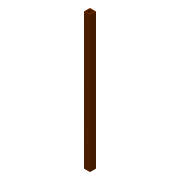
# Autodesk Inventor part: ClawArmBeam
Saved by Autodesk Inventor 2015 (Build 190159000, 159)
## iProperties
Created: 2015-01-13
Part Number: ClawArmBeam
Material: Generic
Document SubType Name: Modeling
Designer: Collin_2
Density: 1 g/cm^3
Appearance: Default
Author: Collin_2
Autodesk Inventor part; units mm, degrees
ref_plane "YZ Plane" through (0, 0, 0) normal (1, 0, 0) x (0, 1, 0)
ref_plane "XZ Plane" through (0, 0, 0) normal (0, 1, 0) x (-1, 0, 0)
ref_plane "XY Plane" through (0, 0, 0) normal (0, 0, 1) x (1, 0, 0)
sketch "Sketch1" plane through (0, 0, 0) normal (0, 1, 0) x (-1, 0, 0)
  line L0 (13.4736, 15.4721) -> (-11.9264, 15.4721)
  line L1 (-11.9264, 15.4721) -> (-11.9264, -9.9279)
  line L2 (-11.9264, -9.9279) -> (13.4736, -9.9279)
  line L3 (13.4736, -9.9279) -> (13.4736, 15.4721)
  point P0 (0, 0)
  dimension "d0" = 25.4
  dimension "d1" = 25.4
  constraints: 8 end point, 2 parallel, 1 horizontal, 1 perpendicular
  measures "d0" distance of L2.end L0.start
  measures "d1" distance of L1.end L2.end
extrude "Extrusion1" add sketch "Sketch1" along normal blind 609.6
shell "Shell1" thickness 3.175 removed faces 1 at (3.4597, 609.6, 7.0054)
sketch "Sketch2" plane through (0, 609.6, 0) normal (0, 1, 0) x (1, 0, 0)
  line L0 (-10.2986, -12.2971) -> (8.7514, -12.2971)
  line L1 (8.7514, -12.2971) -> (8.7514, 6.7529)
  line L2 (8.7514, 6.7529) -> (-10.2986, 6.7529)
  line L3 (-10.2986, 6.7529) -> (-10.2986, -12.2971)
  point P0 (0, 0)
  constraints: 8 end point, 2 parallel, 1 horizontal, 1 perpendicular
extrude "Extrusion2" cut sketch "Sketch2" against normal blind 609.6
sketch "Sketch3" plane through (-13.4736, 0, 15.4721) normal (0, 0, 1) x (1, 0, 0)
  line L0 (38.1, 608.6348) -> (0, 608.6348)
  circle A0 centre (12.7, 12.7) radius 3.3655
  circle A1 centre (12.7, 342.9) radius 3.3655
  circle A2 centre (12.7, 595.9348) radius 3.3655
  line L1 (0, 557.8348) -> (0, 608.6348)
  line L2 (0, 50.8) -> (0, 0)
  line L3 (12.7, 342.9) -> (0, 304.3174) construction
  line L4 (0, 317.5) -> (0, 368.3)
  line L5 (0, 129.921) -> (12.7, 129.921) construction
  circle A3 centre (12.7, 129.921) radius 3.3655
  circle A4 centre (12.7, 174.371) radius 3.3655
  line L6 (9.3413, 197.482) -> (9.3413, 204.213)
  line L7 (16.0611, 204.488) -> (16.0611, 197.3435)
  arc A5 (16.0611, 204.488) -> (9.3413, 204.213) centre (12.6956, 204.488) ccw
  arc A6 (9.3413, 197.482) -> (16.0611, 197.3435) centre (12.6974, 197.231) ccw
  circle A7 centre (12.7, 217.188) radius 3.3655
  line L8 (0, 0) -> (0, 609.6) projected
  point P0 (13.4736, 0)
  dimension "d7" = 38.1
  dimension "d20" = 12.7
  dimension "d29" = 12.7
  dimension "d30" = 6.731
  dimension "d31" = 3.3655
  dimension "d32" = 3.3655
  dimension "d33" = 6.731
  dimension "d34" = 12.7
  dimension "d36" = 90
  dimension "d37" = 90
  dimension "d40" = 478.7138
  dimension "d44" = 404.1468
  dimension "d45" = 411.2913
  dimension "d48" = 434.2638
  dimension "d49" = 50.8
  dimension "d50" = 240.3348
  dimension "d51" = 291.1348
  dimension "d52" = 557.8348
  constraints: 16 end point, 8 centre point, 5 equal radius, 4 point on circle, 2 parallel, 1 coincident, 1 tangent
  measures "d7" distance of L0.start L0.end
  measures "d20" distance from line of L0 A2.centre
  measures "d29" distance of L5.start L5.end
  measures "d30" distance of L6.start L6.end
  measures "d31" radius of A5
  measures "d32" radius of A6
  measures "d33" diameter of A7
  measures "d34" distance of A5.centre A7.centre
  measures "d36" angle of L1 L0
  measures "d37" angle of L4 L0
  measures "d40" distance between parallel lines of L5 L0
  measures "d44" distance from line of L7.start L0
  measures "d45" distance from line of L7.end L0
  measures "d48" distance from line of A4.centre L0
  measures "d49" distance from line of L1.start L0
  measures "d50" distance from line of L4.end L0
  measures "d51" distance from line of L4.start L0
  measures "d52" distance from line of L2.start L0
extrude "Extrusion3" cut sketch "Sketch3" against normal blind 76.2
sketch "Sketch4" plane through (-13.4736, 0, 15.4721) normal (0, 0, 1) x (1, 0, 0)
  line L0 (0, 0) -> (25.4, 0)
  line L1 (25.4, 0) -> (25.4, 25.4)
  line L2 (25.4, 25.4) -> (0, 25.4)
  line L3 (0, 25.4) -> (0, 0)
  point P0 (13.4736, 0)
  dimension "d55" = 25.4
  dimension "d56" = 25.4
  constraints: 8 end point, 2 parallel, 1 horizontal, 1 perpendicular
  measures "d55" distance of L2.end L1.end
  measures "d56" distance of L1.end L0.end
extrude "Extrusion4" cut sketch "Sketch4" against normal blind 25.4
body "Solid1"
